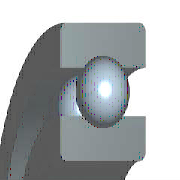
# Autodesk Inventor part: JIS B 1521 SKF - SKF 6012
Saved by Autodesk Inventor 2021 (Build 250183000, 183)
## iProperties
Created: 2020-01-22
Part Number: JIS B 1521 SKF - SKF 6012
Material: Steel, Mild
Description: Single row ball bearings SKF
Document SubType Name: Modeling
Standard: JIS B 1521 SKF
Designer: Eugene Tang
Standard Revision: SKF 2013
Standards Organization: JIS
Language: en-US
Size Designation: SKF 6012
Categories: <MemberInstance><Categories><Category DisplayName="Shaft Parts" InternalName="7f7aeb1f-a693-4053-b835-cee3144e0d98" Mnemonic="SHFT"><Category DisplayName="Bearings" InternalName="242d30a3-7172-44e6-a363-b0a3d8f1b556" Mnemonic="BRNG"><CategoryParameter DisplayName="Width" InternalName="25fc5f6e-338b-4801-b5ed-8959743e396e" Mnemonic="wdth"/><CategoryParameter DisplayName="Size Designation" InternalName="2c4e891a-c8f4-49ed-a5c1-5131476c6feb" Mnemonic="sizedes"/><CategoryParameter DisplayName="Basic Dynamic Load Rating" InternalName="440972dd-7009-4861-bd45-69ffbb461423" Mnemonic="bdynlrat"/><CategoryParameter DisplayName="Shaft Diameter" InternalName="91302473-2833-4451-a660-c5d4a8d6a031" Mnemonic="shaftdia"/><CategoryParameter DisplayName="Touch Angle" InternalName="aa21a452-7974-4a55-b5cf-1c2972de2aea" Mnemonic="TouchAngle"/><CategoryParameter DisplayName="Outer Diameter" InternalName="d441686c-04bd-4681-b674-94fbc173ec23" Mnemonic="outdia"/><Category DisplayName="Ball Bearings" InternalName="9b553946-0899-4a5e-a403-c1d9295e77c1" Mnemonic="BALLBEAR"><CategoryParameter DisplayName="Radial Dynamic Load Factor when Fa/Fr &lt;= e" InternalName="051e59b3-bd55-4dad-8b07-38b5cb912881" Mnemonic="raddynfc1"/><CategoryParameter DisplayName="Basic Static Load Rating" InternalName="0f13fbbf-c511-4d43-b4c7-197b47424baf" Mnemonic="bstatlrat"/><CategoryParameter DisplayName="Exponent for Determining Life" InternalName="3029e2ef-9460-4be8-bdfd-dfe61437473d" Mnemonic="lifeexp"/><CategoryParameter DisplayName="Friction Factor" InternalName="3086b0f2-3d69-46ff-8a75-fe12e395bb47" Mnemonic="fricfct"/><CategoryParameter DisplayName="Min. Shaft Diameter" InternalName="4a5be9bc-ad86-4bf2-8167-102dad5d3e27" Mnemonic="minshaftdia"/><CategoryParameter DisplayName="Axial Dynamic Load Factor when Fa/Fr &gt; e" InternalName="4b6ff741-5956-4a40-80f5-34eb9259f88c" Mnemonic="axdynfc2"/><CategoryParameter DisplayName="Limiting Speed Lubrication Grease" InternalName="5237843b-2c8d-46d3-8227-f3e9dd85a12e" Mnemonic="lubgrsp"/><CategoryParameter DisplayName="Limiting Speed Oil" InternalName="60628548-8907-44dc-8e09-603d72f5766f" Mnemonic="oilspd"/><CategoryParameter DisplayName="Axial Static Load Factor" InternalName="74dbf5e2-8362-409a-802f-3c2235668d99" Mnemonic="axdynfc0"/><CategoryParameter DisplayName="Mass" InternalName="7b80f85c-da81-4dea-b8db-d7c689da91b2" Mnemonic="mass"/><CategoryParameter DisplayName="Radius" InternalName="83352640-dfae-4cba-bc9f-11ecbfb0001c" Mnemonic="rad"/><CategoryParameter DisplayName="Radial Static Load Factor" InternalName="83ce084d-c51e-4598-a871-e8e1e34b26ee" Mnemonic="raddynfc0"/><CategoryParameter DisplayName="Axial Dynamic Load Factor when Fa/Fr &lt;= e" InternalName="ae45a7db-08df-4411-99a8-2f035015bff9" Mnemonic="axdynfc1"/><CategoryParameter DisplayName="Max. Hub Step Diameter" InternalName="b5cf89e0-ca87-439c-b08c-a25e2999ab06" Mnemonic="maxhubdia"/><CategoryParameter DisplayName="Limiting Value for Factor Determination" InternalName="be0ce6fc-cad4-4218-b484-c34dd2571812" Mnemonic="limvalfac"/><CategoryParameter DisplayName="Radial Dynamic Load Factor when Fa/Fr &gt; e" InternalName="e513bdb7-139f-4b3c-af32-49e0ba1226b9" Mnemonic="raddynfc2"/><CategoryParameter DisplayName="Max. Step Fillet Radius" InternalName="f6ce6695-cf2c-4ec9-8d20-66671e0e35a4" Mnemonic="maxstprad"/><Category DisplayName="Deep Groove Ball Bearings" InternalName="6f040212-0f73-4fa8-b5e4-17d6525fdc38" Mnemonic="BBDGBB"/></Category></Category></Category><Category DisplayName="DataType" InternalName="23b78d0f-2648-40c6-8793-ca6db495c9e8" Mnemonic="DATATYPE"><CategoryParameter DisplayName="DisplayName" InternalName="05415f3d-3907-474b-a020-eb9d644f4cf3" Mnemonic="DISPLAYNAME"/><CategoryParameter DisplayName="Standard" InternalName="0c0a119c-1e12-4c84-803f-101930972f5e" Mnemonic="STANDARD"/><CategoryParameter DisplayName="Description" InternalName="13903e3d-64b1-4950-80da-f627842ea37f" Mnemonic="DESCRIPTION"/><CategoryParameter DisplayName="Designation" InternalName="2675968c-4ce5-49e0-a4f5-552d29089031" Mnemonic="DESIGNATION"/><CategoryParameter DisplayName="Default Row" InternalName="2af9ec52-faaa-4026-b378-f9fa4afca842" Mnemonic="DEFAULTROW"/><CategoryParameter DisplayName="Folder Name" InternalName="3f06958e-8713-4116-9be7-ed6184ecc97b" Mnemonic="FOLDERNAME"/><CategoryParameter DisplayName="Revision Guid" InternalName="45a75005-10b1-4dfc-8d6d-dfe629f0b93c" Mnemonic="REVISIONGUID"/><CategoryParameter DisplayName="FileName" InternalName="8b46a4cc-9585-4fed-90c3-899f57e09a73" Mnemonic="FILENAME"/><CategoryParameter DisplayName="StdsOrg" InternalName="8f5914e1-4693-403f-8ab5-d37768198c9d" Mnemonic="STDSORG"/><CategoryParameter DisplayName="Family Version" InternalName="914462f6-6e19-4b14-ba84-155b9680b1d0" Mnemonic="FAMILYREVISION"/><CategoryParameter DisplayName="Standard Revision" InternalName="91d5a463-65c2-4fde-b823-3b7fea5e8e17" Mnemonic="STANDARDREVISION"/><CategoryParameter DisplayName="Member Revision" InternalName="a65d44b9-392f-4f4f-857b-e4b3d54996fe" Mnemonic="MEMBERREVISION"/><CategoryParameter DisplayName="ClipFormat" InternalName="bc51e27b-3422-4e78-93ef-cec197ddf230" Mnemonic="CLIPFORMAT"/><CategoryParameter DisplayName="Manufacturer" InternalName="cd6c7a72-a28a-4e50-99a9-2c7f4e13e5ad" Mnemonic="MANUFACTURER"/><CategoryParameter DisplayName="InternalName" InternalName="cf1d0246-76d9-4b4a-8305-fa0409afb5c1" Mnemonic="INTERNALNAME"/><CategoryParameter DisplayName="IsMetric" InternalName="e2385c5b-1ea4-4823-96a8-8de651266ec3" Mnemonic="ISMETRIC"/><Category DisplayName="Part" InternalName="c0e0b642-3bcb-4cc8-9e80-f96d35c4afa4" Mnemonic="PART"><CategoryParameter DisplayName="Part Number" InternalName="016b6077-bfbe-49bd-92c9-d8d59c39c941" Mnemonic="PARTNUMBER"/><CategoryParameter DisplayName="Stock Number" InternalName="4dba7c1c-e26c-444e-836c-b08b433409a8" Mnemonic="STOCKNUMBER"/><CategoryParameter DisplayName="Material Key" InternalName="5c9a8adb-dd2b-4535-b97f-0a94a95fe41f" Mnemonic="MATERIALKEY"/><CategoryParameter DisplayName="Material" InternalName="818a152a-d3c3-49ca-80ee-df7d91421b8e" Mnemonic="MATERIAL"/></Category></Category><Category DisplayName="Legacy Map DA" InternalName="924fff40-ddd0-4eff-ad42-30e3774ef79e" Mnemonic="LEGACYMAPDA"><CategoryParameter DisplayName="DACookie" InternalName="316934ee-8fe1-4c7a-9c36-f2d79e1add1a" Mnemonic="DACOOKIE"/></Category></Categories><FamilyTemplate Id="N024630"><FamilyTemplateParameters><FamilyTemplateParameter ObjectType="kUserParameterObject" ValueType="xs:double" Id="1" ObjectReferenceKey="Diam"/><FamilyTemplateParameter ObjectType="kUserParameterObject" ValueType="xs:integer" Id="2" ObjectReferenceKey="DD"/><FamilyTemplateParameter ObjectType="kUserParameterObject" ValueType="xs:double" Id="3" ObjectReferenceKey="B"/><FamilyTemplateParameter ObjectType="kUserParameterObject" ValueType="xs:double" Id="4" ObjectReferenceKey="r"/><FamilyTemplateParameter ObjectType="kPropertyObject" ValueType="xs:string" Id="100" ObjectReferenceKey="{32853F0F-3444-11d1-9E93-0060B03C1CA6}" SubObjectId="52"/><FamilyTemplateParameter ObjectType="kPropertyObject" ValueType="xs:string" Id="105" ObjectReferenceKey="{32853F0F-3444-11d1-9E93-0060B03C1CA6}" SubObjectId="5"/><FamilyTemplateParameter ObjectType="kPartComponentDefinitionObject" ValueType="xs:string" Id="110" SubObjectId="Material"/></FamilyTemplateParameters></FamilyTemplate><CategoryParameterMap><ParamToTemplateMap><ParamToTemplate CategoryParameter="//CategoryParameter[@InternalName='05415f3d-3907-474b-a020-eb9d644f4cf3']" ConstantValue="JIS B 1521 SKF"/><ParamToTemplate CategoryParameter="//CategoryParameter[@InternalName='cf1d0246-76d9-4b4a-8305-fa0409afb5c1']" ConstantValue="7AC90127-8084-4CAE-982F-AD5CB6F383C7"/><ParamToTemplate CategoryParameter="//CategoryParameter[@InternalName='3f06958e-8713-4116-9be7-ed6184ecc97b']" ConstantValue="JIS B 1521 SKF (1)"/><ParamToTemplate CategoryParameter="//CategoryParameter[@InternalName='914462f6-6e19-4b14-ba84-155b9680b1d0']" ConstantValue="10"/><ParamToTemplate CategoryParameter="//CategoryParameter[@InternalName='bc51e27b-3422-4e78-93ef-cec197ddf230']" ConstantValue="CF_INVENTOR.STDPARTS"/><ParamToTemplate CategoryParameter="//CategoryParameter[@InternalName='e2385c5b-1ea4-4823-96a8-8de651266ec3']" ConstantValue="true"/><ParamToTemplate CategoryParameter="//CategoryParameter[@InternalName='13903e3d-64b1-4950-80da-f627842ea37f']" ConstantValue="Single row ball bearings"/><ParamToTemplate CategoryParameter="//CategoryParameter[@InternalName='8f5914e1-4693-403f-8ab5-d37768198c9d']" ConstantValue="JIS"/><ParamToTemplate CategoryParameter="//CategoryParameter[@InternalName='0c0a119c-1e12-4c84-803f-101930972f5e']" ConstantValue="JIS B 1521 SKF"/><ParamToTemplate CategoryParameter="//CategoryParameter[@InternalName='cd6c7a72-a28a-4e50-99a9-2c7f4e13e5ad']" TemplateParameter="104"/><ParamToTemplate CategoryParameter="//CategoryParameter[@InternalName='91d5a463-65c2-4fde-b823-3b7fea5e8e17']" ConstantValue="SKF 2013"/><ParamToTemplate CategoryParameter="//CategoryParameter[@InternalName='45a75005-10b1-4dfc-8d6d-dfe629f0b93c']" ConstantValue="dd13a2b2-39d5-48ed-81da-ddf8a2ec956f"/><ParamToTemplate CategoryParameter="//CategoryParameter[@InternalName='2af9ec52-faaa-4026-b378-f9fa4afca842']" ConstantValue="10"/><ParamToTemplate CategoryParameter="//CategoryParameter[@InternalName='8b46a4cc-9585-4fed-90c3-899f57e09a73']" ConstantValue="JIS - SKF 6012"/><ParamToTemplate CategoryParameter="//CategoryParameter[@InternalName='a65d44b9-392f-4f4f-857b-e4b3d54996fe']" ConstantValue="6126F157-EF2A-4942-8221-C124F968C321"/><ParamToTemplate CategoryParameter="//CategoryParameter[@InternalName='0f13fbbf-c511-4d43-b4c7-197b47424baf']" ConstantValue="23200"/><ParamToTemplate CategoryParameter="//CategoryParameter[@InternalName='5237843b-2c8d-46d3-8227-f3e9dd85a12e']" ConstantValue="9500"/><ParamToTemplate CategoryParameter="//CategoryParameter[@InternalName='3086b0f2-3d69-46ff-8a75-fe12e395bb47']" ConstantValue="0.0015"/><ParamToTemplate CategoryParameter="//CategoryParameter[@InternalName='3029e2ef-9460-4be8-bdfd-dfe61437473d']" ConstantValue="3"/><ParamToTemplate CategoryParameter="//CategoryParameter[@InternalName='4a5be9bc-ad86-4bf2-8167-102dad5d3e27']" ConstantValue="66"/><ParamToTemplate CategoryParameter="//CategoryParameter[@InternalName='b5cf89e0-ca87-439c-b08c-a25e2999ab06']" ConstantValue="89"/><ParamToTemplate CategoryParameter="//CategoryParameter[@InternalName='f6ce6695-cf2c-4ec9-8d20-66671e0e35a4']" ConstantValue="1"/><ParamToTemplate CategoryParameter="//CategoryParameter[@InternalName='60628548-8907-44dc-8e09-603d72f5766f']" ConstantValue="15000"/><ParamToTemplate CategoryParameter="//CategoryParameter[@InternalName='83ce084d-c51e-4598-a871-e8e1e34b26ee']" ConstantValue="0.6"/><ParamToTemplate CategoryParameter="//CategoryParameter[@InternalName='74dbf5e2-8362-409a-802f-3c2235668d99']" ConstantValue="0.5"/><ParamToTemplate CategoryParameter="//CategoryParameter[@InternalName='051e59b3-bd55-4dad-8b07-38b5cb912881']" ConstantValue="1"/><ParamToTemplate CategoryParameter="//CategoryParameter[@InternalName='ae45a7db-08df-4411-99a8-2f035015bff9']" ConstantValue="0"/><ParamToTemplate CategoryParameter="//CategoryParameter[@InternalName='2c4e891a-c8f4-49ed-a5c1-5131476c6feb']" ConstantValue="6012"/><ParamToTemplate CategoryParameter="//CategoryParameter[@InternalName='316934ee-8fe1-4c7a-9c36-f2d79e1add1a']" ConstantValue="*JIS~N024630A~SKF 6012*"/><ParamToTemplate CategoryParameter="//CategoryParameter[@InternalName='25fc5f6e-338b-4801-b5ed-8959743e396e']" TemplateParameter="3"/><ParamToTemplate CategoryParameter="//CategoryParameter[@InternalName='d441686c-04bd-4681-b674-94fbc173ec23']" TemplateParameter="2"/><ParamToTemplate CategoryParameter="//CategoryParameter[@InternalName='2675968c-4ce5-49e0-a4f5-552d29089031']" TemplateParameter="100"/><ParamToTemplate CategoryParameter="//CategoryParameter[@InternalName='91302473-2833-4451-a660-c5d4a8d6a031']" TemplateParameter="1"/><ParamToTemplate CategoryParameter="//CategoryParameter[@InternalName='818a152a-d3c3-49ca-80ee-df7d91421b8e']" TemplateParameter="110"/><ParamToTemplate CategoryParameter="//CategoryParameter[@InternalName='016b6077-bfbe-49bd-92c9-d8d59c39c941']" TemplateParameter="105"/><ParamToTemplate CategoryParameter="//CategoryParameter[@InternalName='83352640-dfae-4cba-bc9f-11ecbfb0001c']" TemplateParameter="4"/></ParamToTemplateMap></CategoryParameterMap></MemberInstance>
Mass: 388.526 g
Surface Area: 269.648 cm^2
Volume: 49.4937 cm^3
Density: 7.85 g/cm^3
Appearance: Semi-Polished
IsCustomPart: 0
Author: Eugene Tang
Autodesk Inventor part; units mm, degrees
ref_plane "YZ Plane" through (0, 0, 0) normal (1, 0, 0) x (0, 1, 0)
sketch "Sketch1" plane through (0, 0, 0) normal (0, 0, 1) x (1, 0, 0)
  point P0 (0, 0)
sketch "Sketch2" plane through (0, 0, 0) normal (1, 0, 0) x (0, 1, 0)
  line L0 (30, 18) -> (47.5, 18)
  line L1 (30, 0) -> (30, 18)
  line L2 (47.5, 0) -> (30, 0)
  line L3 (47.5, 18) -> (47.5, 0)
  line L4 (0, 0) -> (0, 20) construction
  line L5 (0, 0) -> (0, 20)
  line L6 (-7.2, 0) -> (43.2, 0) projected
  dimension "d1" = 60
  dimension "d3" = 95
  dimension "d5" = 18
  constraints: 12 end point, 3 vertical, 2 horizontal, 1 collinear, 1 other
  measures "d1" diameter of L0.start L4
  measures "d3" diameter of L0.end L4
  measures "d5" distance of L1.start L0.start
revolve "Revolution1" add sketch "Sketch2" angle 360 about axis through (0, 0, 0) along (0, 0, 1)
ref_plane "WorkPlane3" through (0, 0, 0) normal (0, 0, -1) x (-1, 0, 0)
sketch "Sketch3" plane through (0, 0, 0) normal (1, 0, 0) x (0, 1, 0)
  arc A0 (41.9, 4.8) -> (41.9, 13.2) centre (38.75, 9) ccw
  line L0 (41.9, 18) -> (41.9, 13.2)
  line L1 (35.6, 18) -> (41.9, 18)
  line L2 (35.6, 13.2) -> (35.6, 18)
  arc A1 (35.6, 13.2) -> (35.6, 4.8) centre (38.75, 9) ccw
  line L3 (35.6, 0) -> (35.6, 4.8)
  line L4 (41.9, 0) -> (35.6, 0)
  line L5 (41.9, 4.8) -> (41.9, 0)
  line L6 (47.5, 0) -> (-47.5, 0) construction
  line L7 (47.5, 18) -> (-47.5, 18) construction
  line L8 (0, -42.2904) -> (0, 61.2904)
  line L9 (0, 82.0066) -> (0, -63.0066) projected
  dimension "d9" = 10.5
  dimension "d21" = 35.6
  dimension "d22" = 38.75
  dimension "d23" = 41.9
  constraints: 14 end point, 4 collinear, 4 point on circle, 4 vertical, 2 centre point, 2 concentric, 2 horizontal, 2 point on line
  measures "d9" diameter of A0
  measures "d21" distance between parallel lines of L8 L3
  measures "d22" distance from line of L8 A0.centre
  measures "d23" distance between parallel lines of L8 L5
revolve "Revolution2" cut sketch "Sketch3" angle 360 about axis through (0, 0, -42.2904) along (0, 0, 1)
ref_plane "WorkPlane4" through (0, 0, 18) normal (0, 0, -1) x (-1, 0, 0)
sketch "Sketch4" plane through (0, 0, 18) normal (0, 0, -1) x (-1, 0, 0)
  point P0 (0, 0)
sketch "Sketch5" plane through (0, 0, 0) normal (1, 0, 0) x (0, 1, 0)
  arc A0 (38.75, 3.75) -> (38.75, 14.2501) centre (38.75, 9) ccw
  line L0 (38.75, 3.75) -> (38.75, 14.2501)
  line L1 (41.9, 0) -> (-41.9, 0) construction
  line L2 (38.75, 3.75) -> (38.75, 14.2501)
  arc A1 (41.9, 4.8) -> (41.9, 13.2) centre (38.75, 9) ccw projected
  dimension "d13" = 0
  dimension "d15" = 10.5001
  constraints: 4 end point, 2 point on circle, 1 centre point, 1 concentric, 1 vertical
  measures "d13" horizontal distance of A0.centre L0.start
  measures "d15" diameter of A0
revolve "Revolution3" add sketch "Sketch5" angle 360 about axis through (0, 38.75, 3.75) along (0, 0, 1)
pattern_circular "PolarArray1" count 11 over 360 about axis through (0, 0, 9) along (0, 0, 1) of "Revolution3"
fillet "Fillet1" radius 1.1 4 edges at (0, -47.5, 18) (0, -47.5, 0) (0, -30, 18) (0, -30, 0)
equation "\"d17\" = msp_pocet"
equation "\"d20\" = r"
equation "\"d1\" = Diam"
equation "\"d3\" = DD"
equation "\"d5\" = msp_mdtd2"
equation "\"d9\" = msp_mdtd6"
equation "\"d21\" = 0.5 * msp_d1"
equation "\"d22\" = 0.5 * msp_ds"
equation "\"d23\" = 0.5 * msp_dd1"
equation "\"Diam\" = 60"
equation "\"DD\" = 95"
equation "\"B\" = 18"
equation "\"r\" = 1.1"
equation "\"msp_ds\" = 0.5 * Diam + 0.5 * DD"
equation "\"msp_d0\" = -0.3 * Diam + 0.3 * DD"
equation "\"msp_d1\" = msp_ds - 0.6 * msp_d0"
equation "\"msp_dd1\" = msp_ds + 0.6 * msp_d0"
equation "\"msp_pom\" = 1.5 * msp_ds"
equation "\"msp_mdtd2\" = B"
equation "\"msp_mdtd4\" = msp_ds"
equation "\"msp_mdtd6\" = msp_d0"
equation "\"msp_mdtd7\" = 0.5 * msp_mdtd2"
equation "\"msp_pocet\" = 11.471429"
body "Solid1"
